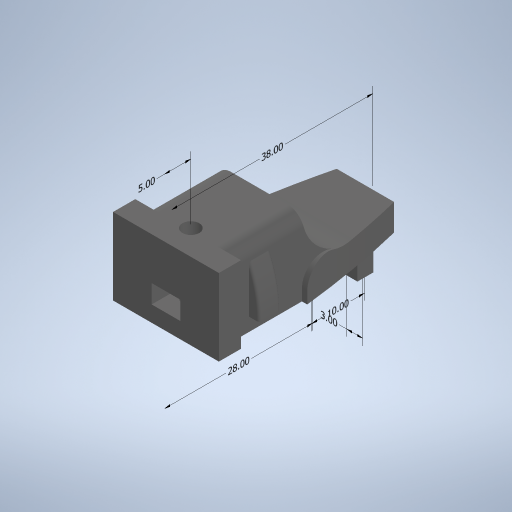
# Autodesk Inventor part: connector_male
Saved by Autodesk Inventor 2024.1 (Build 281209000, 209)
## iProperties
Created: 2025-09-28
Part Number: connector_male
Material: 一般
Document SubType Name: Modeling
Designer: hibik
Density: 1 g/cm^3
Appearance: 既定
Author: hibik
Autodesk Inventor part; units mm, degrees
ref_plane "YZ Plane" through (0, 0, 0) normal (1, 0, 0) x (0, 1, 0)
ref_plane "XZ Plane" through (0, 0, 0) normal (0, 1, 0) x (-1, 0, 0)
ref_plane "XY Plane" through (0, 0, 0) normal (0, 0, 1) x (1, 0, 0)
sketch "スケッチ1" plane through (0, 0, 0) normal (0, 1, 0) x (-1, 0, 0)
  line L0 (10, -0.3) -> (0, -0.3)
  line L1 (0, -0.3) -> (0, -5)
  line L2 (0, -5) -> (10, -5)
  line L3 (10, -5) -> (10, -0.3)
  line L4 (8.5, -5) -> (0, -5)
  line L5 (0, -5) -> (0, -18)
  line L6 (0, -18) -> (8.5, -18)
  line L7 (8.5, -18) -> (8.5, -5)
  line L8 (10, -18) -> (0, -18)
  line L9 (0, -18) -> (0, -28)
  line L10 (0, -28) -> (10, -28)
  line L11 (10, -28) -> (10, -18)
  point P0 (0, 0)
  dimension "d0" = 10
  dimension "d2" = 1.5
  dimension "d3" = 13
  dimension "d34" = 5
  dimension "d35" = 0.3
  constraints: 24 end point, 6 parallel, 4 collinear, 4 perpendicular, 3 horizontal, 2 point on line, 1 coincident
  measures "d0" distance of L0.start L0.end
  measures "d2" distance between parallel lines of L3 L7
  measures "d3" distance of L6.end L4.start
  measures "d34" distance from line of point (0, 0) L2
  measures "d35" distance from line of point (0, 0) L0
extrude "押し出し1" add sketch "スケッチ1" along normal blind 15
sketch "スケッチ3" plane through (-10, 0, -18) normal (0, 0, 1) x (1, 0, 0)
  line L0 (0, 0) -> (1.5, 0) projected
  line L1 (1.5, 0) -> (1.5, 15) projected
  line L2 (0, 15) -> (1.5, 15) projected
  line L3 (0, 0) -> (0, 15) projected
  line L4 (0, 0) -> (10, 0) projected
  line L5 (10, 0) -> (10, 15) projected
  line L6 (0, 15) -> (10, 15) projected
  line L7 (0, 0) -> (0, 15) projected
  circle A0 centre (4.5, 12) radius 3
  circle A1 centre (4.5, 12) radius 2.5
  line L8 (2, 12) -> (2, 0)
  line L9 (4.5, 14.5) -> (10, 14.5)
  point P0 (1.5, 15)
  point P1 (1.5, 0)
  dimension "d6" = 6
  dimension "d7" = 0.5
  constraints: 4 end point, 4 tangent, 2 centre point, 2 perpendicular, 2 point on circle, 2 point on line, 1 coincident
  measures "d6" diameter of A0
  measures "d7" radial gap between concentric circles of A0 A1
extrude "押し出し2" cut sketch "スケッチ3" along normal up to surface (13 mm away) contours L1 A0 L8 L4 | L1 L6 A0 | A0 L9 A1 L8 | L6 L5 L9 A0 picked at (5.4334, 14.5914)
sketch "スケッチ4" plane through (0, 15, 0) normal (0, 1, 0) x (1, 0, 0)
  line L0 (0, 5) -> (-10, 5) projected
  line L1 (-10, 5) -> (-10, 0.3) projected
  line L2 (-10, 0.3) -> (0, 0.3) projected
  line L3 (0, 0.3) -> (0, 5) projected
  point P0 (0, 0)
extrude "押し出し3" cut sketch "スケッチ4" against normal up to surface (0.5 mm away)
sketch "スケッチ5" plane through (-8, 0, -18) normal (-1, 0, 0) x (0, 0, 1)
  line L0 (13, 0) -> (18, 0) projected
  line L1 (13, 0) -> (3, 0)
  line L2 (3, 0) -> (3, 15)
  line L3 (3, 15) -> (13, 15)
  line L4 (13, 15) -> (13, 0)
  line L5 (6, 12) -> (10, 12)
  line L6 (10, 12) -> (10, 2)
  line L7 (10, 2) -> (6, 2)
  line L8 (6, 2) -> (6, 12)
  line L9 (13, 0) -> (0, 0) projected
  point P0 (6.5, 0)
  point P1 (8, 12)
  point P2 (8, 15)
  dimension "d12" = 10
  dimension "d13" = 3
  dimension "d14" = 2
  dimension "d15" = 4
  dimension "d21" = 15
  constraints: 16 end point, 4 parallel, 3 midpoint, 2 horizontal, 2 perpendicular, 1 vertical alignment
  measures "d12" distance of L2.end L3.end
  measures "d13" distance between parallel lines of L3 L5
  measures "d14" distance from line of point (6.5, 0) L7
  measures "d15" distance of L6.end L7.end
  measures "d21" distance of L1.end L2.end
extrude "押し出し4" add sketch "スケッチ5" along normal blind 2 contours L5 L6 L7 L8
sketch "スケッチ6" plane through (-8, 2, -8) normal (0, 0, 1) x (1, 0, 0)
  line L0 (0, 10) -> (0, 0) projected
  line L1 (0, 10) -> (-2, 10) projected
  line L2 (-2, 0) -> (-2, 10) projected
  line L3 (0, 0) -> (-2, 0) projected
  line L4 (0, 0) -> (0, 10) projected
  arc A0 (0, 9.5) -> (-2, 0.5) centre (19.25, 0.5) ccw
  line L5 (-2, 0.5) -> (0, 0.5)
  point P0 (8, -2)
  point P1 (0, 0.5)
  dimension "d22" = 0.5
  dimension "d23" = 0.5
  constraints: 3 point on line, 2 end point, 2 point on circle, 1 centre point, 1 perpendicular, 1 tangent
  measures "d22" distance from line of L1 A0.start
  measures "d23" distance from line of L3 L5.start
extrude "押し出し5" cut sketch "スケッチ6" against normal up to surface (4 mm away) contours L0 A0 L2 L1 | L0 L3 L2 L5
fillet "フィレット1" radius 0.5 2 edges at (-9.494, 7.1098, -12) (-9.494, 7.1098, -8)
mirror "ミラー1" about plane through (0, 0, -0.3) normal (1, 0, 0)
sketch "スケッチ7" plane through (-5.5, 14.5, -5) normal (0, 0, -1) x (-1, 0, 0)
  line L0 (4.5, 0) -> (0, 0) projected
  arc A0 (2.5, -2.5) -> (0, 0) centre (0, -2.5) ccw projected
  line L1 (2.5, -14.5) -> (2.5, -2.5) projected
  line L2 (4.5, -14.5) -> (2.5, -14.5) projected
  line L3 (4.5, -14.5) -> (4.5, 0) projected
  line L4 (-15.5, 0) -> (-11, 0) projected
  line L5 (-15.5, -14.5) -> (-15.5, 0) projected
  line L6 (-15.5, -14.5) -> (-13.5, -14.5) projected
  line L7 (-13.5, -14.5) -> (-13.5, -2.5) projected
  arc A1 (-11, 0) -> (-13.5, -2.5) centre (-11, -2.5) ccw projected
  point P0 (-5.5, -14.5)
extrude "押し出し6" cut sketch "スケッチ7" against normal blind 0.5
sketch "スケッチ8" plane through (-10, 0, -28) normal (0, 0, -1) x (-1, 0, 0)
  line L0 (-20, 0) -> (-20, 15) projected
  line L1 (0, 0) -> (0, 15) projected
  line L2 (-20, 0) -> (0, 0)
  line L3 (0, 0) -> (0, 5)
  line L4 (0, 5) -> (-20, 5)
  line L5 (-20, 5) -> (-20, 0)
  point P0 (-10, 0)
  dimension "d26" = 5
  constraints: 8 end point, 2 parallel, 1 horizontal, 1 perpendicular, 1 point on line
  measures "d26" distance between parallel lines of L2 L4
extrude "押し出し7" add sketch "スケッチ8" along normal blind 10
sketch "スケッチ9" plane through (0, 0, 0) normal (0, -1, 0) x (1, 0, 0)
  line L0 (10, -28) -> (-10, -28) projected
  line L1 (10, -28) -> (10, -38) projected
  line L2 (-10, -38) -> (10, -38) projected
  line L3 (-10, -28) -> (-10, -38) projected
  line L4 (-10, -38) -> (10, -38) projected
  line L5 (1.5, -38) -> (-1.5, -38)
  line L6 (-1.5, -38) -> (-1.5, -28)
  line L7 (-1.5, -28) -> (1.5, -28)
  line L8 (1.5, -28) -> (1.5, -38)
  line L9 (5, -31.5) -> (-5, -31.5)
  line L10 (-5, -31.5) -> (-5, -34.5)
  line L11 (-5, -34.5) -> (5, -34.5)
  line L12 (5, -34.5) -> (5, -31.5)
  point P0 (0, 0)
  point P1 (0, -28)
  point P2 (1.5, -33)
  point P3 (0, -31.5)
  point P4 (5, -33)
  point P5 (1.5, -31.5)
  point P6 (1.5, -28)
  point P7 (-1.5, -31.5)
  point P8 (-1.5, -34.5)
  point P9 (-1.5, -38)
  point P10 (1.5, -34.5)
  dimension "d29" = 3
  dimension "d30" = 3
  constraints: 16 end point, 5 midpoint, 4 parallel, 3 perpendicular, 2 horizontal, 2 point on line, 1 horizontal alignment, 1 vertical alignment
  measures "d29" distance between parallel lines of L6 L8
  measures "d30" distance of L11.end L9.start
extrude "押し出し8" add sketch "スケッチ9" along normal blind 5 contours L8 L9 L6 L0 | L9 L12 L11 L8 | L8 L11 L6 L9 | L2 L6 L11 L8 | L6 L11 L10 L9
sketch "スケッチ11" plane through (-5.5, 14.5, -18) normal (0, 1, 0) x (1, 0, 0)
  line L0 (-8.5, -18) -> (19.5, -18) projected
  line L1 (6.8568, -10.65) -> (8.2135, -13)
  line L2 (8.2135, -13) -> (6.8568, -15.35)
  line L3 (6.8568, -15.35) -> (4.1432, -15.35)
  line L4 (4.1432, -15.35) -> (2.7865, -13)
  line L5 (2.7865, -13) -> (4.1432, -10.65)
  line L6 (4.1432, -10.65) -> (6.8568, -10.65)
  circle A0 centre (5.5, -13) radius 1.6
  line L7 (2.7865, -13) -> (2.7865, -18)
  line L8 (8.2135, -13) -> (8.2135, -18)
  line L9 (-4.5, -17.7) -> (15.5, -17.7) projected
  point P0 (5.5, -18)
  point P1 (2.7865, -17.7)
  point P2 (8.2135, -17.7)
  dimension "d36" = 4.7
  dimension "d37" = 5
  dimension "d38" = 3.2
  constraints: 16 end point, 2 point on line, 2 vertical, 1 centre point, 1 coincident, 1 horizontal, 1 vertical alignment, 13 other
  measures "d36" distance between parallel lines of L6 L3
  measures "d37" distance from line of L0 point (5.5, -13)
  measures "d38" diameter of A0
extrude "押し出し9" cut sketch "スケッチ11" against normal through all contours A0
extrude "押し出し10" cut sketch "スケッチ11" against normal blind 11.5 contours L5 L6 L1 L2 L3 L4
extrude "押し出し11" cut sketch "スケッチ11" against normal up to surface (11.5 mm away) contours L7 L9 L8 L0 | L7 L4 L3 L2 L8 L9
extrude "押し出し12" add sketch "スケッチ11" against normal blind 8 contours L7 L4 L3 L2 L8 L9 | L5 L6 L1 L2 L3 L4
sketch "スケッチ12" plane through (-10, 0, -18) normal (-1, 0, 0) x (0, 0, 1)
  line L0 (-10, 5) -> (-20, 5) projected
  line L1 (-10, 15) -> (0, 15) projected
  line L2 (-10, 5) -> (-10, 15) projected
  arc A0 (-10, 5) -> (0, 14.5) centre (-9.5125, 14.5) ccw
  line L3 (0, 0) -> (0, 15) projected
  line L4 (13.5, 14.5) -> (0, 14.5) projected
  point P0 (18, 0)
  constraints: 2 point on circle, 1 centre point, 1 tangent
extrude "押し出し13" cut sketch "スケッチ12" against normal through all
fillet "フィレット2" radius 4 1 edges at (-7.75, 14.5, -18)
sketch "スケッチ13" plane through (-10, 14.5, -0.3) normal (0, 1, 0) x (1, 0, 0)
  arc A0 (21.586, 79.673) -> (5.1529, 40) centre (157.8276, 0) ccw projected
  arc A1 (46.2266, 111.6009) -> (0, 0) centre (157.8276, 0) ccw projected
  line L0 (0, 27.7) -> (0, 37.7) projected
  line L1 (0, 23.3318) -> (0, 27.7) projected
  line L2 (0, 17.7) -> (0, 23.3318) projected
  line L3 (0, 17.7) -> (2, 17.7) projected
  line L4 (0, 37.7) -> (20, 37.7) projected
  point P0 (10, -0.3)
  point P1 (0.9956, 17.7)
  point P2 (4.5688, 37.7)
extrude "押し出し14" cut sketch "スケッチ13" against normal through all
mirror "ミラー2" about plane through (0, 0, 0) normal (1, 0, 0) of "押し出し14"
equation "\"d22\" = d23"
equation "\"d30\" = d29"
